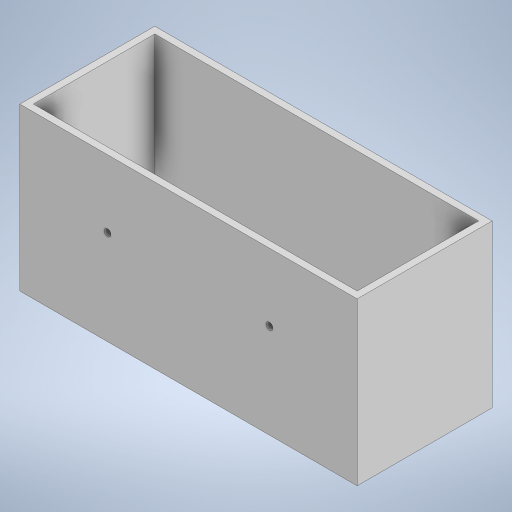
# Autodesk Inventor part: Team29_BaseofBox
Saved by Autodesk Inventor 2023 (Build 270158000, 158)
## iProperties
Created: 2023-02-27
Part Number: Team29_BaseofBox
Material: Generic
Document SubType Name: Modeling
Designer: Fariha
Density: 1 g/cm^3
Appearance: Default
Author: Fariha
Autodesk Inventor part; units mm, degrees
ref_plane "YZ Plane" through (0, 0, 0) normal (1, 0, 0) x (0, 1, 0)
ref_plane "XZ Plane" through (0, 0, 0) normal (0, 1, 0) x (-1, 0, 0)
ref_plane "XY Plane" through (0, 0, 0) normal (0, 0, 1) x (1, 0, 0)
sketch "Sketch1" plane through (0, 0, 0) normal (0, 1, 0) x (-1, 0, 0)
  line L0 (125, 50) -> (-125, 50)
  line L1 (-125, 50) -> (-125, -50)
  line L2 (-125, -50) -> (125, -50)
  line L3 (125, -50) -> (125, 50)
  line L4 (120, 45) -> (-120, 45)
  line L5 (-120, 45) -> (-120, -45)
  line L6 (-120, -45) -> (120, -45)
  line L7 (120, -45) -> (120, 45)
  point P0 (0, 0)
  dimension "d0" = 250
  dimension "d1" = 100
  dimension "d2" = 50
  dimension "d3" = 125
  dimension "d4" = 5
  dimension "d5" = 5
  dimension "d6" = 5
  dimension "d7" = 5
  constraints: 16 end point, 4 parallel, 2 horizontal, 2 perpendicular
  measures "d0" distance of L2.end L1.end
  measures "d1" distance of L1.end L0.end
  measures "d2" distance from line of point (0, 0) L0
  measures "d3" distance from line of point (0, 0) L3
  measures "d4" distance between parallel lines of L3 L7
  measures "d5" distance between parallel lines of L0 L4
  measures "d6" distance between parallel lines of L2 L6
  measures "d7" distance between parallel lines of L1 L5
extrude "Extrusion1" add sketch "Sketch1" along normal blind 5 contours L7 L6 L5 L4
sketch "Sketch2" plane through (0, 0, 0) normal (0, -1, 0) x (1, 0, 0)
  line L0 (-125, -50) -> (125, -50)
  line L1 (125, -50) -> (125, 50)
  line L2 (125, 50) -> (-125, 50)
  line L3 (-125, 50) -> (-125, -50)
  line L4 (-120, -45) -> (-120, 45) projected
  line L5 (120, 45) -> (120, -45) projected
  line L6 (-120, 45) -> (120, 45) projected
  line L7 (120, -45) -> (-120, -45) projected
  line L8 (-120, -45) -> (-120, 45) projected
  line L9 (120, 45) -> (120, -45) projected
  line L10 (-120, -45) -> (120, -45)
  line L11 (120, -45) -> (120, 45)
  line L12 (120, 45) -> (-120, 45)
  line L13 (-120, 45) -> (-120, -45)
  point P0 (0, 0)
  dimension "d10" = 5
  dimension "d11" = 5
  dimension "d12" = 5
  dimension "d13" = 5
  constraints: 16 end point, 4 parallel, 2 horizontal, 2 perpendicular
  measures "d10" distance between parallel lines of L3 L4
  measures "d11" distance between parallel lines of L1 L5
  measures "d12" distance between parallel lines of L6 L2
  measures "d13" distance between parallel lines of L0 L7
extrude "Extrusion2" add sketch "Sketch2" against normal blind 120
sketch "Sketch4" plane through (-125, 0, 50) normal (0, 0, 1) x (1, 0, 0)
  circle A0 centre (65, 70) radius 2.5
  circle A1 centre (185, 70) radius 2.5
  line L0 (250, 0) -> (0, 0) projected
  line L1 (250, 0) -> (250, 120) projected
  point P0 (125, 0)
  point P1 (250, 60)
  dimension "d16" = 5
  dimension "d17" = 5
  dimension "d18" = 70
  dimension "d19" = 70
  dimension "d20" = 120
  dimension "d21" = 65
  constraints: 2 centre point, 1 midpoint
  measures "d16" diameter of A0
  measures "d17" diameter of A1
  measures "d18" distance from line of L0 A1.centre
  measures "d19" distance from line of L0 A0.centre
  measures "d20" distance of A1.centre A0.centre
  measures "d21" horizontal distance of point (250, 60) A1.centre
extrude "Extrusion3" cut sketch "Sketch4" against normal blind 5
body "Solid1"
